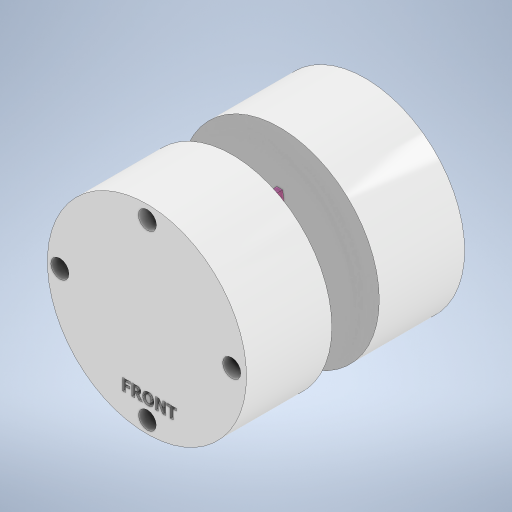
# Autodesk Inventor part: spine
Saved by Autodesk Inventor 2024 (Build 280153000, 153)
## iProperties
Created: 2024-08-07
Part Number: spine
Material: Generic
Document SubType Name: Modeling
Designer: maint
Density: 1 g/cm^3
Appearance: Default
Author: maint
Autodesk Inventor part; units mm, degrees
ref_plane "YZ Plane" through (0, 0, 0) normal (1, 0, 0) x (0, 1, 0)
ref_plane "XZ Plane" through (0, 0, 0) normal (0, 1, 0) x (-1, 0, 0)
ref_plane "XY Plane" through (0, 0, 0) normal (0, 0, 1) x (1, 0, 0)
sketch "Sketch1" plane through (0, 0, 0) normal (0, 0, 1) x (1, 0, 0)
  circle A0 centre (0, 0) radius 52.5
  dimension "d2" = 105
  constraints: 1 centre point, 1 coincident
  measures "d2" diameter of A0
extrude "Extrusion1" add sketch "Sketch1" along normal blind 45
sketch "Sketch2" plane through (0, 0, 45) normal (0, 0, 1) x (1, 0, 0)
  line L0 (0, 24.7077) -> (1.5126, 24.7077)
  line L1 (1.5126, 24.7077) -> (2.8012, 16.3312)
  line L2 (2.8012, 16.3312) -> (3.2694, 13.2883)
  line L3 (3.2694, 13.2883) -> (7.3116, 7.8474)
  line L4 (7.3116, 7.8474) -> (10.1038, 6.1291)
  line L5 (10.1038, 6.1291) -> (13.6509, 3.9463)
  line L6 (13.6509, 3.9463) -> (17.5995, 1.5164)
  line L7 (17.5995, 1.5164) -> (20.0636, 0)
  line L8 (20.0636, 0) -> (21.2368, -1.5791)
  line L9 (21.2368, -1.5791) -> (21.2368, -5.1469)
  line L10 (21.2368, -5.1469) -> (18.4846, -7.1916)
  line L11 (18.4846, -7.1916) -> (15.6252, -9.3159)
  line L12 (15.6252, -9.3159) -> (13.6509, -10.7827)
  line L13 (13.6509, -10.7827) -> (13.2405, -11.0876)
  line L14 (13.2405, -11.0876) -> (8.4381, -11.0876)
  line L15 (8.4381, -11.0876) -> (7.165, -12.0335)
  line L16 (7.165, -12.0335) -> (3.005, -12.6735)
  line L17 (3.005, -12.6735) -> (0, -14.263)
  line L18 (0, -24.3011) -> (0, 28.1525)
  line L19 (0, 24.7077) -> (-1.5126, 24.7077)
  line L20 (-1.5126, 24.7077) -> (-2.8012, 16.3312)
  line L21 (-2.8012, 16.3312) -> (-3.2694, 13.2883)
  line L22 (-3.2694, 13.2883) -> (-7.3116, 7.8474)
  line L23 (-7.3116, 7.8474) -> (-10.1038, 6.1291)
  line L24 (-10.1038, 6.1291) -> (-13.6509, 3.9463)
  line L25 (-13.6509, 3.9463) -> (-17.5995, 1.5164)
  line L26 (-17.5995, 1.5164) -> (-20.0636, 0)
  line L27 (-20.0636, 0) -> (-21.2368, -1.5791)
  line L28 (-21.2368, -1.5791) -> (-21.2368, -5.1469)
  line L29 (-21.2368, -5.1469) -> (-18.4846, -7.1916)
  line L30 (-18.4846, -7.1916) -> (-15.6252, -9.3159)
  line L31 (-15.6252, -9.3159) -> (-13.6509, -10.7827)
  line L32 (-13.6509, -10.7827) -> (-13.2405, -11.0876)
  line L33 (-13.2405, -11.0876) -> (-8.4381, -11.0876)
  line L34 (-8.4381, -11.0876) -> (-7.165, -12.0335)
  line L35 (-7.165, -12.0335) -> (-3.005, -12.6735)
  line L36 (-3.005, -12.6735) -> (0, -14.263)
  point P0 (0, 0)
  constraints: 74 end point, 18 point on line, 17 symmetric about line, 3 parallel, 3 perpendicular, 1 horizontal, 1 vertical
extrude "Extrusion2" add sketch "Sketch2" along normal blind 10
sketch "Sketch3" plane through (0, 0, 55) normal (0, 0, 1) x (1, 0, 0)
  line L0 (-1.5126, 24.7077) -> (1.5126, 24.7077) projected
  line L1 (0, 24.7077) -> (1.5382, 23.5426)
  line L2 (1.5382, 23.5426) -> (3.0757, 13.5489)
  line L3 (3.2694, 13.2883) -> (1.5126, 24.7077) projected
  line L4 (7.3116, 7.8474) -> (3.2694, 13.2883) projected
  line L5 (3.0757, 13.5489) -> (7.3116, 7.8474)
  line L6 (7.3116, 7.8474) -> (12.2469, 6.433)
  line L7 (12.2469, 6.433) -> (14.8387, 4.47)
  line L8 (14.8387, 4.47) -> (15.2998, 1.473)
  line L9 (15.2998, 1.473) -> (14.8387, -0.1358)
  line L10 (14.8387, -0.1358) -> (15.8688, -2.2258)
  line L11 (15.8688, -2.2258) -> (15.3595, -5.7473)
  line L12 (15.3595, -5.7473) -> (15.3595, -8.4068)
  line L13 (15.3595, -8.4068) -> (14.7752, -9.7874)
  line L14 (14.7752, -9.7874) -> (14.0661, -10.7236)
  line L15 (14.0661, -10.7236) -> (11.7001, -11.0876)
  line L16 (13.2405, -11.0876) -> (8.4381, -11.0876) projected
  line L17 (11.7001, -11.0876) -> (8.4381, -11.0876)
  line L18 (8.4381, -11.0876) -> (7.8373, -11.7077)
  line L19 (0, -14.263) -> (3.005, -12.6735) projected
  line L20 (7.8373, -11.7077) -> (3.005, -12.6735)
  line L21 (3.005, -12.6735) -> (0, -14.263)
  line L22 (0, 29.9699) -> (0, -23.5626) construction
  line L23 (0, 24.7077) -> (-1.5382, 23.5426)
  line L24 (-1.5382, 23.5426) -> (-3.0757, 13.5489)
  line L25 (-7.3116, 7.8474) -> (-3.2694, 13.2883)
  line L26 (-3.0757, 13.5489) -> (-7.3116, 7.8474)
  line L27 (-7.3116, 7.8474) -> (-12.2469, 6.433)
  line L28 (-12.2469, 6.433) -> (-14.8387, 4.47)
  line L29 (-14.8387, 4.47) -> (-15.2998, 1.473)
  line L30 (-15.2998, 1.473) -> (-14.8387, -0.1358)
  line L31 (-14.8387, -0.1358) -> (-15.8688, -2.2258)
  line L32 (-15.8688, -2.2258) -> (-15.3595, -5.7473)
  line L33 (-15.3595, -5.7473) -> (-15.3595, -8.4068)
  line L34 (-15.3595, -8.4068) -> (-14.7752, -9.7874)
  line L35 (-14.7752, -9.7874) -> (-14.0661, -10.7236)
  line L36 (-14.0661, -10.7236) -> (-11.7001, -11.0876)
  line L37 (-11.7001, -11.0876) -> (-8.4381, -11.0876)
  line L38 (-8.4381, -11.0876) -> (-7.8373, -11.7077)
  line L39 (0, -14.263) -> (-3.005, -12.6735)
  line L40 (-7.8373, -11.7077) -> (-3.005, -12.6735)
  point P0 (0, 0)
  point P1 (-13.2405, -11.0876)
  constraints: 72 end point, 18 symmetric about line, 6 point on line, 3 parallel, 3 perpendicular, 2 collinear, 2 vertical, 1 horizontal, 1 midpoint
extrude "Extrusion3" add sketch "Sketch3" along normal blind 5 contours L1 L2 L5 L4 L6 L7 L8 L9 L10 L11 L12 L13 L14 L15 L16 L18 L20 L19 L39 L40 L38 L37 L36 L35 L34 L33 L32 L31 L30 L29 L28 L27 L25 L26 L24 L23
sketch "Sketch4" plane through (0, 0, 60) normal (0, 0, 1) x (1, 0, 0)
  line L0 (0, -14.263) -> (3.005, -12.6735) projected
  line L1 (0, -14.263) -> (3.005, -12.6735)
  line L2 (3.005, -12.6735) -> (7.165, -12.0335)
  line L3 (7.165, -12.0335) -> (8.332, -10.9167)
  line L4 (8.332, -10.9167) -> (13.2141, -11.4765)
  line L5 (13.2141, -11.4765) -> (21.0207, -5.0806)
  line L6 (21.0207, -5.0806) -> (21.0207, -1.2876)
  line L7 (13.2405, -11.0876) -> (8.4381, -11.0876) projected
  line L8 (21.0207, -1.2876) -> (19.8662, 0.1215)
  line L9 (15.0519, 3.0841) -> (7.3116, 7.8474) projected
  line L10 (19.8662, 0.1215) -> (7.3116, 7.8474)
  line L11 (7.3116, 7.8474) -> (3.2694, 13.2883)
  line L12 (3.2694, 13.2883) -> (1.5126, 24.7077) projected
  line L13 (3.2694, 13.2883) -> (1.5126, 24.7077)
  line L14 (0, 24.7077) -> (-1.5126, 24.7077) projected
  line L15 (1.5126, 24.7077) -> (0, 24.7077)
  line L16 (0.0748, -21.3754) -> (0.0748, 33.5667)
  line L17 (0.1496, -14.263) -> (-2.8553, -12.6735)
  line L18 (0.1496, -14.263) -> (-2.8553, -12.6735)
  line L19 (-2.8553, -12.6735) -> (-7.0154, -12.0335)
  line L20 (-7.0154, -12.0335) -> (-8.1824, -10.9167)
  line L21 (-8.1824, -10.9167) -> (-13.0645, -11.4765)
  line L22 (-13.0645, -11.4765) -> (-20.871, -5.0806)
  line L23 (-20.871, -5.0806) -> (-20.871, -1.2876)
  line L24 (-13.0908, -11.0876) -> (-8.2885, -11.0876)
  line L25 (-20.871, -1.2876) -> (-19.7166, 0.1215)
  line L26 (-14.9023, 3.0841) -> (-7.162, 7.8474)
  line L27 (-19.7166, 0.1215) -> (-7.162, 7.8474)
  line L28 (-7.162, 7.8474) -> (-3.1197, 13.2883)
  line L29 (-3.1197, 13.2883) -> (-1.3629, 24.7077)
  line L30 (-3.1197, 13.2883) -> (-1.3629, 24.7077)
  line L31 (-1.3629, 24.7077) -> (0.1496, 24.7077)
  point P0 (0, 0)
  point P1 (0.0748, -14.2234)
  constraints: 54 end point, 15 symmetric about line, 3 collinear, 2 perpendicular, 2 point on line, 1 vertical
extrude "Extrusion4" add sketch "Sketch4" along normal blind 10
sketch "Sketch6" plane through (0, 0, 70) normal (0, 0, 1) x (1, 0, 0)
  circle A0 centre (0, 0) radius 52.5
  constraints: 1 centre point, 1 coincident
extrude "Extrusion5" add sketch "Sketch6" along normal blind 45
sketch "Sketch7" plane through (0, 0, 115) normal (0, 0, 1) x (1, 0, 0)
  line L0 (0.2372, -52.4995) -> (0.2372, 52.4995)
  circle A0 centre (0, 0) radius 52.5 projected
  line L1 (52.5, 0) -> (-52.5, 0)
  circle A1 centre (0.2372, 45.3054) radius 4.7809
  circle A2 centre (0.2372, -46.017) radius 4.6603
  circle A3 centre (-45.8984, 0) radius 4.7809
  circle A4 centre (44.7124, 0) radius 4.7809
  line L2 (-13.4647, -32.9709) -> (12.2158, -32.9709) construction
  line L3 (12.2158, -32.9709) -> (12.2158, -38.1893) construction
  line L4 (12.2158, -38.1893) -> (-13.4647, -38.1893) construction
  line L5 (-13.4647, -38.1893) -> (-13.4647, -32.9709) construction
  line L6 (-8.7488, -34.2611) -> (-11.3094, -34.2611)
  line L7 (-11.3094, -34.2611) -> (-11.3094, -35.4129)
  line L8 (-11.3094, -35.4129) -> (-8.9515, -35.4129)
  line L9 (-8.9515, -35.4129) -> (-8.9515, -36.5746)
  line L10 (-8.9515, -36.5746) -> (-11.3094, -36.5746)
  line L11 (-11.3094, -36.5746) -> (-11.3094, -39.1994)
  line L12 (-11.3094, -39.1994) -> (-12.832, -39.1994)
  line L13 (-12.832, -39.1994) -> (-12.832, -33.0994)
  line L14 (-12.832, -33.0994) -> (-8.7488, -33.0994)
  line L15 (-8.7488, -33.0994) -> (-8.7488, -34.2611)
  line L16 (-2.3226, -39.1994) -> (-4.1862, -39.1994)
  line L17 (-4.1862, -39.1994) -> (-5.8817, -36.9601)
  line L18 (-5.8817, -36.9601) -> (-6.4354, -36.9601)
  line L19 (-6.4354, -36.9601) -> (-6.4354, -39.1994)
  line L20 (-6.4354, -39.1994) -> (-7.9579, -39.1994)
  line L21 (-7.9579, -39.1994) -> (-7.9579, -33.0994)
  line L22 (-7.9579, -33.0994) -> (-5.506, -33.0994)
  spline S0 degree 2 poles (-5.506, -33.0994) (-4.9969, -33.0994) (-4.2455, -33.228) (-3.9242, -33.4257) knots 0 0 0 1 2 2 2
  spline S1 degree 2 poles (-3.9242, -33.4257) (-3.5979, -33.6333) (-3.2123, -34.2809) (-3.2123, -34.7752) knots 0 0 0 1 2 2 2
  spline S2 degree 2 poles (-3.2123, -34.7752) (-3.2123, -35.4722) (-3.8451, -36.3472) (-4.374, -36.6042) knots 0 0 0 1 2 2 2
  line L23 (-4.374, -36.6042) -> (-2.3226, -39.1994)
  spline S3 degree 2 poles (-4.7843, -34.968) (-4.7843, -34.7357) (-4.9623, -34.4045) (-5.1649, -34.3155) knots 0 0 0 1 2 2 2
  spline S4 degree 2 poles (-5.1649, -34.3155) (-5.3083, -34.2562) (-5.6593, -34.2216) (-5.9213, -34.2216) knots 0 0 0 1 2 2 2
  line L24 (-5.9213, -34.2216) -> (-6.4354, -34.2216)
  line L25 (-6.4354, -34.2216) -> (-6.4354, -35.8627)
  line L26 (-6.4354, -35.8627) -> (-5.9954, -35.8627)
  spline S5 degree 2 poles (-5.9954, -35.8627) (-5.679, -35.8627) (-5.2292, -35.7836) (-5.076, -35.6601) knots 0 0 0 1 2 2 2
  spline S6 degree 2 poles (-5.076, -35.6601) (-4.9277, -35.5414) (-4.7843, -35.2251) (-4.7843, -34.968) knots 0 0 0 1 2 2 2
  spline S7 degree 2 poles (3.6835, -36.1494) (3.6835, -37.6324) (2.1017, -39.328) (0.7274, -39.328) knots 0 0 0 1 2 2 2
  spline S8 degree 2 poles (0.7274, -39.328) (-0.6517, -39.328) (-2.2237, -37.6127) (-2.2237, -36.1494) knots 0 0 0 1 2 2 2
  spline S9 degree 2 poles (-2.2237, -36.1494) (-2.2237, -34.6813) (-0.6517, -32.9709) (0.7274, -32.9709) knots 0 0 0 1 2 2 2
  spline S10 degree 2 poles (0.7274, -32.9709) (2.1017, -32.9709) (3.6835, -34.6714) (3.6835, -36.1494) knots 0 0 0 1 2 2 2
  spline S11 degree 2 poles (2.1017, -36.1494) (2.1017, -35.6007) (1.8792, -34.8345) (1.6864, -34.5923) knots 0 0 0 1 2 2 2
  spline S12 degree 2 poles (1.6864, -34.5923) (1.4937, -34.3402) (0.9993, -34.1227) (0.7324, -34.1227) knots 0 0 0 1 2 2 2
  spline S13 degree 2 poles (0.7324, -34.1227) (0.4506, -34.1227) (-0.0091, -34.3254) (-0.2217, -34.5824) knots 0 0 0 1 2 2 2
  spline S14 degree 2 poles (-0.2217, -34.5824) (-0.4095, -34.8197) (-0.6418, -35.6057) (-0.6418, -36.1494) knots 0 0 0 1 2 2 2
  spline S15 degree 2 poles (-0.6418, -36.1494) (-0.6418, -36.713) (-0.4194, -37.4545) (-0.2266, -37.7066) knots 0 0 0 1 2 2 2
  spline S16 degree 2 poles (-0.2266, -37.7066) (-0.0338, -37.9587) (0.4655, -38.1762) (0.7324, -38.1762) knots 0 0 0 1 2 2 2
  spline S17 degree 2 poles (0.7324, -38.1762) (1.0043, -38.1762) (1.5085, -37.9439) (1.6914, -37.6967) knots 0 0 0 1 2 2 2
  spline S18 degree 2 poles (1.6914, -37.6967) (1.8891, -37.4298) (2.1017, -36.7229) (2.1017, -36.1494) knots 0 0 0 1 2 2 2
  line L27 (9.8181, -39.1994) -> (8.345, -39.1994)
  line L28 (8.345, -39.1994) -> (5.992, -34.9482)
  line L29 (5.992, -34.9482) -> (5.992, -39.1994)
  line L30 (5.992, -39.1994) -> (4.5931, -39.1994)
  line L31 (4.5931, -39.1994) -> (4.5931, -33.0994)
  line L32 (4.5931, -33.0994) -> (6.4715, -33.0994)
  line L33 (6.4715, -33.0994) -> (8.4192, -36.5943)
  line L34 (8.4192, -36.5943) -> (8.4192, -33.0994)
  line L35 (8.4192, -33.0994) -> (9.8181, -33.0994)
  line L36 (9.8181, -33.0994) -> (9.8181, -39.1994)
  line L37 (12.2304, -39.1994) -> (12.2304, -34.2611)
  line L38 (12.2304, -34.2611) -> (10.4261, -34.2611)
  line L39 (10.4261, -34.2611) -> (10.4261, -33.0994)
  line L40 (10.4261, -33.0994) -> (15.5672, -33.0994)
  line L41 (15.5672, -33.0994) -> (15.5672, -34.2611)
  line L42 (15.5672, -34.2611) -> (13.7629, -34.2611)
  line L43 (13.7629, -34.2611) -> (13.7629, -39.1994)
  line L44 (13.7629, -39.1994) -> (12.2304, -39.1994)
  constraints: 4 centre point, 4 end point, 4 point on circle, 4 point on line, 1 horizontal, 1 vertical, 2 other
sketch "Sketch8" plane through (0, 0, 0) normal (0, 0, -1) x (-1, 0, 0)
  circle A0 centre (34.5127, -31.7849) radius 4.3738
  circle A1 centre (-34.0383, -31.7849) radius 4.2762
  circle A2 centre (-34.2755, 30.8361) radius 4.5131
  circle A3 centre (34.5127, 30.8361) radius 4.3738
  point P0 (0, 0)
  constraints: 4 centre point
extrude "Extrusion6" cut sketch "Sketch8" against normal blind 10
extrude "Extrusion7" cut sketch "Sketch7" against normal blind 10 contours A2 L0 | L0 A2 | A3 L1 | L1 A3 | A4 L1 | L1 A4 | S8 S9 L0 S13 S14 S15 S16 | L0 S16 S17 S18 S11 S12 S13 S9 S10 S7 S8 | A1 L0 | L0 A1 | L6 L7 L8 L9 L10 L11 L12 L13 L14 L15 | L16 L17 L18 L19 L20 L21 L22 S0 S1 S2 L23 | L27 L28 L29 L30 L31 L32 L33 L34 L35 L36 | L37 L38 L39 L40 L41 L42 L43 L44
body "Solid1"
